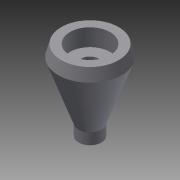
# Autodesk Inventor part: Stack
Saved by Autodesk Inventor 2015 (Build 190159000, 159)
## iProperties
Created: 2018-03-26
Part Number: Stack
Material: Generic
Document SubType Name: Modeling
Designer: Administrator
Density: 1 g/cm^3
Appearance: Default
Author: Administrator
Autodesk Inventor part; units mm, degrees
ref_plane "YZ Plane" through (0, 0, 0) normal (1, 0, 0) x (0, 1, 0)
ref_plane "XZ Plane" through (0, 0, 0) normal (0, 1, 0) x (-1, 0, 0)
ref_plane "XY Plane" through (0, 0, 0) normal (0, 0, 1) x (1, 0, 0)
sketch "Sketch1" plane through (0, 0, 0) normal (0, 0, 1) x (1, 0, 0)
  line L0 (15.875, 44.45) -> (17.5765, 38.1)
  line L1 (17.5765, 38.1) -> (6.35, 6.35)
  line L2 (6.35, 6.35) -> (6.35, 0)
  line L3 (6.35, 0) -> (0, 0)
  line L4 (0, 0) -> (0, 44.45)
  line L5 (15.875, 44.45) -> (0, 44.45)
  dimension "d0" = 6.35
  dimension "d1" = 6.35
  dimension "d2" = 44.45
  dimension "d3" = 75
  dimension "d4" = 38.1
  constraints: 12 end point, 2 perpendicular, 1 vertical
  measures "d0" distance of L1.end L2.end
  measures "d1" distance of L2.end L3.end
  measures "d2" distance of L3.end L4.end
  measures "d3" angle of L5 L0
  measures "d4" distance from line of L3 L0.end
revolve "Revolution1" add sketch "Sketch1" angle 360 about axis through (0, 0, 0) along (0, 1, 0)
sketch "Sketch2" plane through (0, 44.45, 0) normal (0, 1, 0) x (1, 0, 0)
  point P0 (0, 0)
  point P1 (0, 0)
  constraints: 1 coincident
hole "Hole1" at (0, 44.45, 0) direction (0, -1, 0) diameter 9.525 depth 38.1 tip angle 118 counterbore diameter 22.225 counterbore depth 9.525
chamfer "Chamfer1" distance 0.254 angle 45 1 edges at (-6.35, 0, 0)
body "Solid1"
